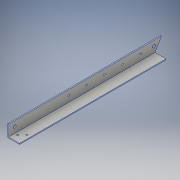
# Autodesk Inventor part: CLB_084_ClimberMountTopAngle
Saved by Autodesk Inventor 2018.3 (Build 223284000, 284)
## iProperties
Created: 2020-02-22
Part Number: CLB_084_ClimberMountTopAngle
Material: Aluminum 6061
Document SubType Name: Modeling
Designer: 22perngrac
Density: 2.7 g/cm^3
Appearance: Aluminum - Flat
Mass: 291.92 g
Surface Area: 721.162 cm^2
Volume: 108.119 cm^3
Author: 22perngrac
Autodesk Inventor part; units mm, degrees
ref_plane "YZ Plane" through (0, 0, 0) normal (1, 0, 0) x (0, 1, 0)
ref_plane "XZ Plane" through (0, 0, 0) normal (0, 1, 0) x (-1, 0, 0)
ref_plane "XY Plane" through (0, 0, 0) normal (0, 0, 1) x (1, 0, 0)
sketch "Sketch1" plane through (0, 0, 0) normal (0, 0, 1) x (1, 0, 0)
  line L0 (0, 0) -> (0, 38.1)
  line L1 (0, 38.1) -> (3.175, 38.1)
  line L2 (3.175, 38.1) -> (3.175, 3.175)
  line L3 (3.175, 3.175) -> (38.1, 3.175)
  line L4 (38.1, 3.175) -> (38.1, 0)
  line L5 (38.1, 0) -> (0, 0)
  dimension "d0" = 38.1
  dimension "d1" = 3.175
  constraints: 12 end point, 6 perpendicular, 1 parallel, 1 vertical
  measures "d0" distance of L4.end L0.start
  measures "d1" distance of L3.end L4.end
extrude "Extrusion1" add sketch "Sketch1" along normal blind 485.775
sketch "Sketch4" plane through (3.175, 3.175, 0) normal (1, 0, 0) x (0, 0, -1)
  line L0 (0, 0) -> (-485.775, 0) projected
  line L1 (0, -3.175) -> (0, 34.925) projected
  line L2 (0, 34.925) -> (-26.0631, -10.2176)
  line L3 (-26.0631, -10.2176) -> (14.7874, -10.2176)
  line L4 (14.7874, -10.2176) -> (14.7874, 34.925)
  line L5 (14.7874, 34.925) -> (0, 34.925)
  line L6 (-20.164, 0) -> (29.2522, 0)
  dimension "d6" = 60
  constraints: 10 end point, 3 perpendicular, 3 point on line
  measures "d6" angle of L6 L2
extrude "Extrusion2" cut sketch "Sketch4" along normal mid plane 476.25
sketch "Sketch5" plane through (3.175, 3.175, 485.775) normal (1, 0, 0) x (0, 0, -1)
  line L0 (0, 0) -> (0, 34.925) projected
  line L1 (465.611, 0) -> (0, 0) projected
  line L2 (465.611, 0) -> (485.775, 34.925) projected
  line L3 (485.775, 34.925) -> (0, 34.925) projected
  line L4 (471.1103, 34.925) -> (450.9463, 0)
  point P0 (485.775, -3.175)
  point P1 (19.05, 19.05)
  point P2 (461.9449, 19.05)
  dimension "d9" = 19.05
  dimension "d10" = 19.05
  dimension "d11" = 12.7
  constraints: 3 point on line, 2 end point, 1 horizontal alignment, 1 parallel
  measures "d9" distance from line of L0 point (19.05, 19.05)
  measures "d10" distance from line of L1 point (19.05, 19.05)
  measures "d11" distance between parallel lines of L4 L2
hole "Hole1" at (3.175, 22.225, 466.725) at (3.175, 22.225, 23.8301) direction (-1, 0, 0) diameter 9.525 end through all
sketch "Sketch6" plane through (3.175, 3.175, 485.775) normal (0, 1, 0) x (1, 0, 0)
  line L0 (0, 485.775) -> (0, 0) projected
  line L1 (34.925, 0) -> (0, 0) projected
  line L2 (34.925, 465.611) -> (34.925, 0) projected
  point P0 (-3.175, 485.775)
  point P1 (23.3172, 34.7472)
  point P2 (8.9154, 19.4564)
  dimension "d20" = 8.9154
  dimension "d21" = 19.4564
  dimension "d22" = 11.6078
  dimension "d23" = 34.7472
  measures "d20" distance from line of L0 point (8.915, 19.456)
  measures "d21" distance from line of L1 point (8.915, 19.456)
  measures "d22" distance from line of L2 point (23.317, 34.747)
  measures "d23" distance from line of L1 point (23.317, 34.747)
hole "Hole2" at (26.4922, 3.175, 451.0278) at (12.0904, 3.175, 466.3186) direction (0, -1, 0) diameter 5.1054 end through all
sketch "Sketch7" plane through (3.175, 3.175, 485.775) normal (1, 0, 0) x (0, 0, -1)
  circle A0 centre (19.05, 19.05) radius 4.7625 projected
  line L0 (0, 0) -> (0, 34.925) projected
  point P0 (485.775, -3.175)
  point P1 (190.5, 19.05)
  point P2 (247.65, 19.05)
  point P3 (304.8, 19.05)
  point P4 (361.95, 19.05)
  point P5 (419.1, 19.05)
  dimension "d31" = 190.5
  dimension "d32" = 57.15
  dimension "d35" = 57.15
  dimension "d45" = 57.15
  dimension "d46" = 57.15
  constraints: 5 horizontal alignment
  measures "d31" distance from line of point (190.5, 19.05) L0
  measures "d32" distance of point (247.65, 19.05) point (190.5, 19.05)
  measures "d35" distance of point (361.95, 19.05) point (304.8, 19.05)
  measures "d45" distance of point (304.8, 19.05) point (247.65, 19.05)
  measures "d46" distance of point (419.1, 19.05) point (361.95, 19.05)
hole "Hole3" at (3.175, 22.225, 295.275) at (3.175, 22.225, 238.125) at (3.175, 22.225, 180.975) at (3.175, 22.225, 123.825) at (3.175, 22.225, 66.675) direction (-1, 0, 0) diameter 5.1054 end through all clearance for "Flat Head Machine Screw (82)" size "#10" standard "Ansi Unified Screw Threads"
body "Solid1"
